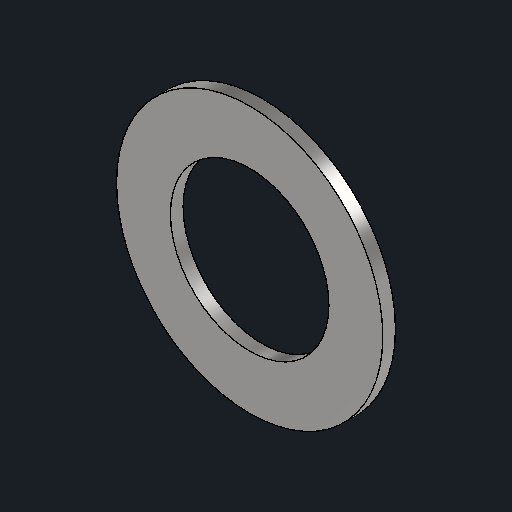
# Autodesk Inventor part: Washer
Saved by Autodesk Inventor 2026.2 (Build 302298000, 298)
## iProperties
Created: 2015-04-29
Part Number: Washer
Material: Stainless Steel
Document SubType Name: Modeling
Designer: Philip
Density: 8 g/cm^3
Appearance: Semi-Polished
Author: Philip
Autodesk Inventor part; units mm, degrees
ref_plane "YZ Plane" through (0, 0, 0) normal (1, 0, 0) x (0, 1, 0)
ref_plane "XZ Plane" through (0, 0, 0) normal (0, 1, 0) x (-1, 0, 0)
ref_plane "XY Plane" through (0, 0, 0) normal (0, 0, 1) x (1, 0, 0)
sketch "Sketch1" plane through (0, 0, 0) normal (0, 0, 1) x (1, 0, 0)
  circle A0 centre (0, 0) radius 6.6675
  circle A1 centre (0, 0) radius 3.9688
  dimension "d0" = 13.335
  dimension "d1" = 7.9375
  constraints: 2 centre point, 2 coincident
  measures "d0" diameter of A0
  measures "d1" diameter of A1
extrude "Extrusion1" add sketch "Sketch1" along normal blind 0.635
body "Solid1"
